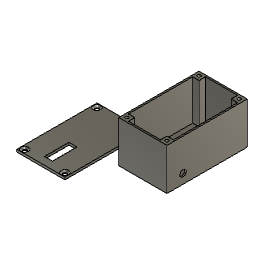
Curtain Opener Box v17 (Autodesk Fusion 360 design; units mm, degrees)
Autodesk Fusion 360 part; units mm, degrees
sketch "Lid" plane through (0, 0, 0) normal (0, 0, 1) x (1, 0, 0)
  line L0 (13.1446, 57.9272) -> (73.1446, 57.9272)
  line L1 (73.1446, 57.9272) -> (73.1446, -42.0728)
  line L2 (73.1446, -42.0728) -> (13.1446, -42.0728)
  line L3 (13.1446, -42.0728) -> (13.1446, 57.9272)
  line L4 (38.1446, -2.0728) -> (48.1446, -2.0728)
  line L5 (48.1446, -2.0728) -> (48.1446, -32.5728)
  line L6 (48.1446, -32.5728) -> (38.1446, -32.5728)
  line L7 (38.1446, -32.5728) -> (38.1446, -2.0728)
  line L8 (43.1446, 57.9272) -> (43.1446, -42.0728) construction
  line L9 (13.1446, 7.9272) -> (73.1446, 7.9272) construction
  dimension "d1" = 60
  dimension "d2" = 100
  dimension "d3" = 10
  dimension "d4" = 30.5
  dimension "d5" = 25
  dimension "d63" = 60
  constraint horizontal L0
  constraint vertical L1
  constraint horizontal L2
  constraint vertical L3
  constraint horizontal L4
  constraint vertical L5
  constraint horizontal L6
  constraint vertical L7
  constraint midpoint L0 L8.start
  constraint midpoint L2 L8.end
  constraint midpoint L3 L9.start
  constraint midpoint L1 L9.end
  measures "d1" distance of L0.start L0.end
  measures "d2" distance of L0.start L2.end
  measures "d3" distance of L4.start L4.end
  measures "d4" distance of L4.start L6.end
  measures "d5" distance of L3 L7
  measures "d63" distance of L0 L4
extrude "Extrude6" add sketch "Lid" along normal blind 2 makes body 1
sketch "Body" plane through (0, 0, 2) normal (0, 0, 1) x (-1, 0, 0)
  line L0 (-48.1446, 32.5728) -> (-38.1446, 32.5728)
  line L1 (-38.1446, 32.5728) -> (-38.1446, 2.0728)
  line L2 (-38.1446, 2.0728) -> (-48.1446, 2.0728)
  line L3 (-48.1446, 2.0728) -> (-48.1446, 32.5728)
  line L4 (-13.1446, 42.0728) -> (-73.1446, 42.0728)
  line L5 (-73.1446, 42.0728) -> (-73.1446, -57.9272)
  line L6 (-73.1446, -57.9272) -> (-13.1446, -57.9272)
  line L7 (-13.1446, -57.9272) -> (-13.1446, 42.0728)
  line L8 (-93.4333, -104.757) -> (-153.4333, -104.757)
  line L9 (-153.4333, -104.757) -> (-153.4333, -4.757)
  line L10 (-153.4333, -4.757) -> (-93.4333, -4.757)
  line L11 (-93.4333, -4.757) -> (-93.4333, -104.757)
  line L12 (-143.4333, -6.757) -> (-103.4333, -6.757)
  line L13 (-95.5059, -14.757) -> (-95.5059, -94.757)
  line L14 (-103.4333, -102.757) -> (-143.4333, -102.757)
  line L15 (-151.5059, -94.757) -> (-151.5059, -14.757)
  line L16 (-93.4333, -104.757) -> (-103.4333, -104.757)
  line L17 (-103.4333, -102.757) -> (-103.4333, -94.757)
  line L18 (-103.4333, -94.757) -> (-95.5059, -94.757)
  line L19 (-93.4333, -94.757) -> (-93.4333, -104.757)
  line L20 (-153.4333, -104.757) -> (-143.4333, -104.757)
  line L21 (-143.4333, -102.757) -> (-143.4333, -94.757)
  line L22 (-143.4333, -94.757) -> (-151.5059, -94.757)
  line L23 (-153.4333, -94.757) -> (-153.4333, -104.757)
  line L24 (-93.4333, -4.757) -> (-103.4333, -4.757)
  line L25 (-103.4333, -6.757) -> (-103.4333, -14.757)
  line L26 (-103.4333, -14.757) -> (-95.5059, -14.757)
  line L27 (-93.4333, -14.757) -> (-93.4333, -4.757)
  line L28 (-153.4333, -4.757) -> (-143.4333, -4.757)
  line L29 (-143.4333, -6.757) -> (-143.4333, -14.757)
  line L30 (-143.4333, -14.757) -> (-151.5059, -14.757)
  line L31 (-153.4333, -14.757) -> (-153.4333, -4.757)
  line L32 (-123.4383, -84.9681) -> (-123.9383, -84.9678)
  line L33 (-125.4374, -83.4669) -> (-125.4353, -79.9669)
  line L34 (-123.4383, -84.9681) -> (-122.9481, -84.9716)
  line L35 (-121.4374, -83.4725) -> (-121.4354, -79.9693)
  arc A0 (-122.9481, -84.9716) -> (-121.4374, -83.4725) centre (-122.9374, -83.4716) ccw
  arc A1 (-125.4374, -83.4669) -> (-123.9383, -84.9678) centre (-123.9374, -83.4678) ccw
  arc A2 (-121.4354, -79.9693) -> (-125.4353, -79.9669) centre (-123.4333, -76.504) ccw
  line L36 (-121.4354, -79.9693) -> (-125.4353, -79.9669) construction
  line L37 (-121.4354, -44.9693) -> (-125.4353, -44.9669) construction
  line L38 (-121.4374, -48.4725) -> (-121.4354, -44.9693)
  line L39 (-125.4374, -48.4669) -> (-125.4353, -44.9669)
  arc A3 (-122.9481, -49.9716) -> (-121.4374, -48.4725) centre (-122.9374, -48.4716) ccw
  arc A4 (-125.4374, -48.4669) -> (-123.9383, -49.9678) centre (-123.9374, -48.4678) ccw
  line L40 (-123.4383, -49.9681) -> (-122.9481, -49.9716)
  arc A5 (-121.4354, -44.9693) -> (-125.4353, -44.9669) centre (-123.4333, -41.504) ccw
  line L41 (-123.4383, -49.9681) -> (-123.9383, -49.9678)
  point P0 (-125.4383, -84.9669)
  point P1 (-121.4383, -84.9823)
  point P2 (-125.4383, -49.9669)
  point P3 (-121.4383, -49.9823)
  dimension "d8" = 60
  dimension "d9" = 100
  dimension "d11" = 10
  dimension "d12" = 10
  dimension "d13" = 10
  dimension "d14" = 10
  dimension "d15" = 10
  dimension "d16" = 10
  dimension "d17" = 10
  dimension "d18" = 10
  dimension "d19" = 8
  dimension "d21" = 2
  dimension "d22" = 2
  dimension "d23" = 1.5
  dimension "d24" = 1.5
  dimension "d26" = 30
  dimension "d27" = 5
  dimension "d30" = 8
  dimension "d31" = 2
  dimension "d32" = 2
  dimension "d33" = 1.5
  dimension "d34" = 1.5
  dimension "d35" = 5
  constraint horizontal L8
  constraint vertical L9
  constraint horizontal L10
  constraint vertical L11
  constraint horizontal L16
  constraint vertical L17
  constraint horizontal L18
  constraint vertical L19
  constraint horizontal L20
  constraint vertical L21
  constraint horizontal L22
  constraint vertical L23
  constraint horizontal L24
  constraint vertical L25
  constraint horizontal L26
  constraint vertical L27
  constraint horizontal L28
  constraint vertical L29
  constraint horizontal L30
  constraint vertical L31
  constraint parallel L10 L12
  constraint parallel L11 L13
  constraint parallel L8 L14
  constraint parallel L9 L15
  constraint perpendicular L32 L33
  constraint perpendicular L32 L35
  constraint coincident P1 L34
  constraint coincident P1 L35
  constraint tangent L34 A0
  constraint tangent L35 A0
  constraint coincident P0 L32
  constraint coincident P0 L33
  constraint tangent L32 A1
  constraint tangent L33 A1
  constraint perpendicular L35 L36
  constraint perpendicular L39 L41
  constraint perpendicular L38 L41
  constraint coincident P3 L40
  constraint coincident P3 L38
  constraint tangent A3 L40
  constraint tangent L38 A3
  constraint coincident P2 L41
  constraint coincident P2 L39
  constraint tangent A4 L41
  constraint tangent L39 A4
  constraint perpendicular L37 L38
  measures "d8" distance of L8.start L8.end
  measures "d9" distance of L8.start L10.end
  measures "d11" distance of L8.start L16.end
  measures "d12" distance of L8.start L19.start
  measures "d13" distance of L8.end L20.end
  measures "d14" distance of L8.end L23.start
  measures "d15" distance of L10.end L24.end
  measures "d16" distance of L10.end L27.start
  measures "d17" distance of L9.end L28.end
  measures "d18" distance of L9.end L31.start
  measures "d19" diameter of A2
  measures "d21" distance of L32.start P0
  measures "d22" distance of L32.start P1
  measures "d23" radius of A0
  measures "d24" radius of A1
  measures "d26" distance of L11 A2.centre
  measures "d27" distance of L32.start L36
  measures "d30" diameter of A5
  measures "d31" distance of P2 L40.start
  measures "d32" distance of P3 L40.start
  measures "d33" radius of A3
  measures "d34" radius of A4
  measures "d35" distance of L40.start L37
extrude "Extrude4" add sketch "Body" along normal blind 52 separate body contours L8 L9 L10 L11 L16 L19 L20 L23 L24 L27 L28 L31 makes body 2
extrude "Extrude5" add sketch "Body" along normal blind 2 contours L12 L13 L14 L15 L17 L18 L21 L22 L25 L26 L29 L30 bodies 2
hole "Hole1" at (98.4333, 99.757, 54) direction (0, 0, -1) diameter 4 depth 16 tip angle 118 bodies 2
ref_plane "WorkPlane1" through (123.4333, 54.757, 28) normal (0, -1, 0) x (1, 0, 0)
ref_plane "WorkPlane2" through (123.4333, 54.757, 28) normal (-1, 0, 0) x (0, -1, 0)
mirror "Mirror1" about plane through (123.4333, 54.757, 28) normal (0, -1, 0) of "Hole1"
mirror "Mirror2" about plane through (123.4333, 54.757, 28) normal (-1, 0, 0) of "Hole1"
mirror "Mirror3" about plane through (123.4333, 54.757, 28) normal (-1, 0, 0) of "Mirror1"
extrude "Extrude8" add 1 faces at (41.478, 37.9272, 2) along direction (0, 0, 1) blind 1 on bodies 1 bodies 1
hole "Hole2" at (123.4333, 104.757, 14) direction (0, -1, 0) diameter 8 depth 3 tip angle 118 bodies 2
hole "Hole3" at (153.4333, 24.757, 14) direction (-1, 0, 0) diameter 8 depth 3 tip angle 118 bodies 2
hole "Hole6" at (18.1446, 52.9272, 3) direction (0, 0, -1) diameter 5 depth 16 tip angle 118 countersink diameter 9.2 countersink angle 90 bodies 1
ref_plane "WorkPlane5" through (43.1446, 7.9272, 1.5) normal (-1, 0, 0) x (0, -1, 0)
hole "Hole7" at (18.1446, -37.0728, 3) direction (0, 0, -1) diameter 5 depth 16 tip angle 118 countersink diameter 9.2 countersink angle 90 bodies 1
hole "Hole8" at (68.1446, -37.0728, 3) direction (0, 0, -1) diameter 5 depth 16 tip angle 118 countersink diameter 9.2 countersink angle 90 bodies 1
hole "Hole9" at (68.1446, 52.9272, 3) direction (0, 0, -1) diameter 5 depth 16 tip angle 118 countersink diameter 9.2 countersink angle 90 bodies 1
delete_face "DeleteFace2" 1 faces at (19.0644, 56.9569, 2.5333) on bodies 1
hole "Hole10" at (38.1446, 52.9272, 3) direction (0, 0, -1) diameter 5 depth 16 tip angle 118 countersink diameter 9.2 countersink angle 90 bodies 1
delete_face "DeleteFace4" 1 faces at (18.3935, 50.4397, 1) on bodies 1
delete_face "DeleteFace5" 1 faces at (34.7295, 55.2556, 2.5333) on bodies 1
delete_face "DeleteFace6" 1 faces at (38.2692, 50.4303, 2) on bodies 1
hole "Hole11" at (18.1446, 52.9272, 3) direction (0, 0, -1) diameter 5 depth 16 tip angle 118 countersink diameter 9.2 countersink angle 90 bodies 1
mirror "Mirror7" [suppressed]
extrude "Extrude7" [suppressed]
ref_plane "WorkPlane3" through (43.1446, 7.9272, 1.5) normal (0, -1, 0) x (1, 0, 0)
ref_plane "WorkPlane4" through (43.1446, 7.9272, 1.5) normal (-1, 0, 0) x (0, -1, 0)
mirror "Mirror4" [suppressed]
mirror "Mirror5" [suppressed]
mirror "Mirror6" [suppressed]
hole "Hole5" [suppressed]
equation "d5 = ( d1 / 2 ) - d3 / 2"
named bodies: "Box", "Lid"
